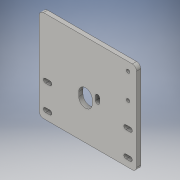
# Autodesk Inventor part: vrRig_v8_projMount01
Saved by Autodesk Inventor 2016 (Build 200138000, 138)
## iProperties
Created: 2018-01-13
Part Number: vrRig_v8_projMount01
Material: Generic
Document SubType Name: Modeling
Designer: harveylab
Density: 1 g/cm^3
Appearance: Default
Author: harveylab
Autodesk Inventor part; units mm, degrees
ref_plane "YZ Plane" through (0, 0, 0) normal (1, 0, 0) x (0, 1, 0)
ref_plane "XZ Plane" through (0, 0, 0) normal (0, 1, 0) x (-1, 0, 0)
ref_plane "XY Plane" through (0, 0, 0) normal (0, 0, 1) x (1, 0, 0)
sketch "Sketch1" plane through (0, 0, 0) normal (0, 0, 1) x (1, 0, 0)
  line L0 (73.2079, 137.9474) -> (121.0158, 137.9474)
  line L1 (133.7158, 0) -> (73.2079, 0)
  line L2 (73.2079, 137.9474) -> (25.4, 137.9474)
  line L3 (25.4, 0) -> (73.2079, 0)
  line L4 (121.0158, 137.9474) -> (140.0658, 137.9474)
  arc A0 (146.4158, 131.5974) -> (140.0658, 137.9474) centre (140.0658, 131.5974) ccw
  line L5 (146.4158, 131.5974) -> (146.4158, 6.35)
  line L6 (25.4, 0) -> (6.35, 0)
  arc A1 (0, 6.35) -> (6.35, 0) centre (6.35, 6.35) ccw
  line L7 (0, 6.35) -> (0, 131.5974)
  arc A2 (6.35, 137.9474) -> (0, 131.5974) centre (6.35, 131.5974) ccw
  line L8 (6.35, 137.9474) -> (25.4, 137.9474)
  line L9 (140.0658, 0) -> (133.7158, 0)
  arc A3 (140.0658, 0) -> (146.4158, 6.35) centre (140.0658, 6.35) ccw
  arc A4 (9.525, 53.975) -> (9.525, 47.625) centre (9.525, 50.8) ccw
  arc A5 (15.875, 47.625) -> (15.875, 53.975) centre (15.875, 50.8) ccw
  line L10 (9.525, 53.975) -> (15.875, 53.975)
  line L11 (9.525, 47.625) -> (15.875, 47.625)
  arc A6 (9.525, 15.875) -> (9.525, 9.525) centre (9.525, 12.7) ccw
  arc A7 (15.875, 9.525) -> (15.875, 15.875) centre (15.875, 12.7) ccw
  line L12 (9.525, 15.875) -> (15.875, 15.875)
  line L13 (9.525, 9.525) -> (15.875, 9.525)
  arc A8 (130.5408, 53.975) -> (130.5408, 47.625) centre (130.5408, 50.8) ccw
  arc A9 (136.8908, 47.625) -> (136.8908, 53.975) centre (136.8908, 50.8) ccw
  line L14 (130.5408, 53.975) -> (136.8908, 53.975)
  line L15 (130.5408, 47.625) -> (136.8908, 47.625)
  arc A10 (130.5408, 15.875) -> (130.5408, 9.525) centre (130.5408, 12.7) ccw
  arc A11 (136.8908, 9.525) -> (136.8908, 15.875) centre (136.8908, 12.7) ccw
  line L16 (130.5408, 15.875) -> (136.8908, 15.875)
  line L17 (130.5408, 9.525) -> (136.8908, 9.525)
  arc A12 (84.5988, 62.6476) -> (90.9488, 62.6476) centre (87.7738, 62.6476) ccw
  arc A13 (90.9488, 68.9976) -> (84.5988, 68.9976) centre (87.7738, 68.9976) ccw
  line L18 (84.5988, 62.6476) -> (84.5988, 68.9976)
  line L19 (90.9488, 62.6476) -> (90.9488, 68.9976)
  circle A14 centre (133.7158, 125.2474) radius 2.54
  circle A15 centre (133.7158, 87.1474) radius 2.54
  arc A16 (79.7508, 61.6154) -> (59.4308, 61.6154) centre (69.5908, 61.6154) ccw
  arc A17 (59.4308, 55.2654) -> (79.7508, 55.2654) centre (69.5908, 55.2654) ccw
  line L20 (79.7508, 55.2654) -> (79.7508, 61.6154)
  line L21 (59.4308, 61.6154) -> (59.4308, 55.2654)
  point P0 (0, 0)
  constraints: 44 end point, 32 point on circle, 18 centre point
extrude "Extrusion1" add sketch "Sketch1" along normal blind 6.35
body "Solid1"
